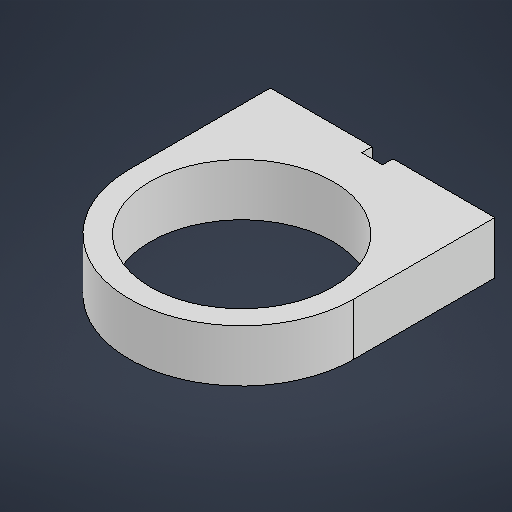
# Autodesk Inventor part: PLATE,BEARING,BLOCK
Saved by Autodesk Inventor 2026.1 (Build 301233020, 233B)
## iProperties
Created: 2026-03-30
Part Number: PLATE,BEARING,BLOCK
Material: Generic
Document SubType Name: Modeling
Designer: Owen L
Density: 1 g/cm^3
Appearance: Default
Author: Owen L
Autodesk Inventor part; units mm, degrees
ref_plane "YZ Plane" through (0, 0, 0) normal (1, 0, 0) x (0, 1, 0)
ref_plane "XZ Plane" through (0, 0, 0) normal (0, 1, 0) x (-1, 0, 0)
ref_plane "XY Plane" through (0, 0, 0) normal (0, 0, 1) x (1, 0, 0)
sketch "Sketch1" plane through (0, 0, 0) normal (0, 1, 0) x (-1, 0, 0)
  circle A0 centre (0, 0) radius 11.1125
  line L0 (13.6525, -17.145) -> (-13.6525, -17.145)
  arc A1 (13.6525, 0) -> (-13.6525, 0) centre (0, 0) ccw
  line L1 (13.6525, 0) -> (13.6525, -17.145)
  line L2 (-13.6525, -17.145) -> (-13.6525, 0)
  dimension "d0" = 22.225
  dimension "d1" = 17.145
  dimension "d2" = 2.54
  constraints: 6 end point, 2 centre point, 2 coincident, 2 point on circle, 2 tangent, 2 vertical, 1 horizontal
  measures "d0" diameter of A0
  measures "d1" distance from line of point (0, 0) L0
  measures "d2" radial gap between concentric circles of A1 A0
extrude "Extrusion1" add sketch "Sketch1" along normal blind 6.35
sketch "Sketch2" plane through (13.6525, 0, -17.145) normal (0, 0, -1) x (-1, 0, 0)
  line L0 (0, 0) -> (27.305, 0) projected
  line L1 (0, 0) -> (0, 6.35) projected
  line L2 (27.305, 0) -> (27.305, 6.35) projected
  point P0 (13.6525, 0)
  point P1 (4.7625, 3.175)
  point P2 (22.5425, 3.175)
  dimension "d5" = 3.175
  dimension "d6" = 4.7625
  dimension "d7" = 4.7625
  constraints: 1 horizontal alignment
  measures "d5" distance from line of L0 point (4.763, 3.175)
  measures "d6" distance from line of L1 point (4.763, 3.175)
  measures "d7" distance from line of L2 point (22.543, 3.175)
hole "Hole1" at (8.89, 3.175, -17.145) at (-8.89, 3.175, -17.145) direction (0, 0, 1) diameter 3.683 depth 6.35 tip angle 118 thread size "10-24 UNC" class "2B" standard "ANSI Unified Screw Threads"
sketch "Sketch3" plane through (0, 6.35, 0) normal (0, 1, 0) x (1, 0, 0)
  line L0 (-1.27, 18.415) -> (1.27, 18.415)
  line L1 (1.27, 18.415) -> (1.27, 15.875)
  line L2 (1.27, 15.875) -> (-1.27, 15.875)
  line L3 (-1.27, 15.875) -> (-1.27, 18.415)
  line L4 (13.6525, 17.145) -> (-13.6525, 17.145) projected
  line L5 (-1.27, 18.415) -> (1.27, 15.875) construction
  line L6 (1.27, 18.415) -> (-1.27, 15.875) construction
  point P0 (0, 0)
  point P1 (0, 17.145)
  point P2 (1.27, 17.145)
  point P3 (-1.27, 17.145)
  dimension "d15" = 2.54
  dimension "d16" = 2.54
  constraints: 12 end point, 3 midpoint, 2 parallel, 1 horizontal, 1 perpendicular
  measures "d15" distance of L1.end L2.end
  measures "d16" distance of L0.end L1.end
extrude "Extrusion2" cut sketch "Sketch3" against normal through all contours L4 L1 L2 L3
equation "\"d7\" = d6"
body "Solid1"
